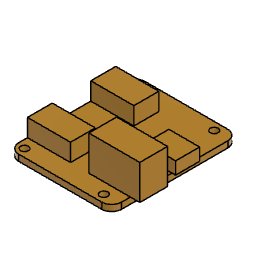
MCP73871 Solar Charger Controller (Autodesk Fusion 360 design; units mm, degrees)
Autodesk Fusion 360 part; units mm, degrees
sketch "Sketch1" plane through (0, 0, 0) normal (0, 0, 1) x (1, 0, 0)
  line L0 (0, 0) -> (33.02, 0)
  line L1 (33.02, 0) -> (33.02, 40.64)
  line L2 (33.02, 40.64) -> (0, 40.64)
  line L3 (0, 40.64) -> (0, 0)
  line L4 (0, 40.64) -> (2.54, 40.64)
  circle A0 centre (2.54, 38.1) radius 1.27
  line L5 (0, 40.64) -> (33.02, 0) construction
  line L6 (33.02, 40.64) -> (0, 0) construction
  line L7 (16.51, 20.32) -> (0, 20.32) construction
  line L8 (16.51, 20.32) -> (16.51, 40.64) construction
  circle A1 centre (2.54, 2.54) radius 1.27
  line L9 (30.46, 38.1) -> (33.02, 38.1) construction
  line L10 (33.02, 38.1) -> (27.94, 38.1) construction
  circle A2 centre (27.94, 38.1) radius 1.27
  circle A3 centre (27.94, 2.54) radius 1.27
  line L11 (0, 40.64) -> (2.54, 40.64)
  line L12 (2.54, 40.64) -> (2.54, 38.1) construction
  line L13 (2.54, 38.1) -> (0, 38.1) construction
  line L14 (0, 38.1) -> (0, 40.64)
  line L15 (27.94, 38.1) -> (33.02, 38.1) construction
  line L16 (33.02, 38.1) -> (33.02, 40.64)
  line L17 (33.02, 40.64) -> (27.94, 40.64)
  line L18 (27.94, 40.64) -> (27.94, 38.1) construction
  line L19 (27.94, 2.54) -> (33.02, 2.54) construction
  line L20 (33.02, 2.54) -> (33.02, 0)
  line L21 (33.02, 0) -> (27.94, 0)
  line L22 (27.94, 0) -> (27.94, 2.54) construction
  line L23 (2.54, 2.54) -> (0, 2.54) construction
  line L24 (0, 2.54) -> (0, 0)
  line L25 (0, 0) -> (2.54, 0)
  line L26 (2.54, 0) -> (2.54, 2.54) construction
  dimension "d1" = 33.02
  dimension "d2" = 40.64
  dimension "d3" = 2.54
  dimension "d5" = 2.54
  dimension "d10" = 5.08
  dimension "d11" = 2.54
  dimension "d16" = 2.54
  constraint horizontal L0
  constraint vertical L1
  constraint horizontal L2
  constraint vertical L3
  constraint coincident L0.start L3.end
  constraint perpendicular L3 L4
  constraint midpoint L5 L7.start
  constraint midpoint L3 L7.end
  constraint midpoint L2 L8.end
  constraint symmetric A0 L7 A1
  constraint coincident L1 L9.end
  constraint perpendicular L1 L9
  constraint parallel L9 L10
  constraint coincident L10.end A2.centre
  constraint symmetric L7 A2 A3
  constraint horizontal L11
  constraint vertical L12
  constraint horizontal L13
  constraint vertical L14
  constraint coincident A0.centre L12.end
  constraint equal L12 L13
  constraint horizontal L15
  constraint vertical L16
  constraint horizontal L17
  constraint vertical L18
  constraint horizontal L19
  constraint vertical L20
  constraint horizontal L21
  constraint vertical L22
  constraint coincident A3.centre L19.start
  constraint horizontal L23
  constraint vertical L24
  constraint horizontal L25
  constraint vertical L26
  constraint coincident A1.centre L23.start
  measures "d1" distance of L0.start L0.end
  measures "d2" distance of L0.start L2.end
  measures "d3" distance of L2.end L4.end
  measures "d5" diameter of A0
  measures "d10" distance of L9.end L10.end
  measures "d11" diameter of A2
  measures "d16" distance of L10.end L17.end
extrude "Extrude1" add sketch "Sketch1" along normal blind 2 contours L0 L1 L2 L3 L4 L11 L14 L16 L17 L20 L21 L24 L25 | A2 | A3 makes body 1
extrude "Extrude2" cut sketch "Sketch1" along normal blind 8.89 contours A2 | A3 bodies 1
fillet "Fillet2" radius 3.175 tangency weight 0.91341 4 edges at (0, 0, 1) (0, 40.64, 1) (33.02, 0, 1) (33.02, 40.64, 1) on bodies 1
ref_plane "WorkPlane1" through (12.7, 20.32, 1) normal (1, 0, 0) x (0, 1, 0)
ref_plane "WorkPlane2" through (16.51, 20.32, 1) normal (0, -1, 0) x (1, 0, 0)
split "Split1" by plane through (12.7, 20.32, 1) normal (1, 0, 0) bodies 1 makes body 2 at (17.5161, 25.9157, 2)
move_body "Move1" bodies 2 to x (1, 0, 0) y (0, 1, 0) z (0, 0, 1) at (7.62, 0, 0)
extrude "Extrude3" add 1 faces at (20.32, 13.5467, 0.6667) along direction (-1, 0, 0) blind 0.19 on bodies 2 bodies 2
move_body "Align1" bodies 1 to x (1, 0, 0) y (0, 1, 0) z (0, 0, 1) at (7.43, 0, 0)
combine "Combine1" operation add target body 1 tool bodies 2
split "Split2" by plane through (16.51, 20.32, 1) normal (0, -1, 0) bodies 1 makes body 3 at (27.6127, 14.7243, 0)
move_body "Move2" bodies 1 to x (1, 0, 0) y (0, 1, 0) z (0, 0, 1) at (0, 15.24, 0)
extrude "Extrude4" add 1 faces at (18.5, 35.56, 1.3333) along direction (0, -1, 0) blind 0.07 on bodies 1 bodies 1
move_body "Align2" bodies 1 to x (1, 0, 0) y (0, 1, 0) z (0, 0, 1) at (0, -15.17, 0)
combine "Combine2" operation add target body 3 tool bodies 1
sketch "Sketch2" plane through (0, 0, 2) normal (0, 0, 1) x (-1, 0, 0)
  circle A0 centre (-35.56, -38.17) radius 1.27
  circle A1 centre (-9.97, -38.17) radius 1.27
  line L0 (-7.43, -37.535) -> (-7.43, -3.175)
  spline S0 degree 3 poles (-10.605, 0) (-10.2204, 0) (-9.8384, -0.0835) (-9.079, -0.3997) (-8.7103, -0.6502) (-8.0884, -1.2692) (-7.8353, -1.6389) (-7.5148, -2.4023) (-7.43, -2.7873) (-7.43, -3.175) knots 0 0 0 0 0.115379 0.115379 0.246087 0.246087 0.377441 0.377441 0.493755 0.493755 0.493755 0.493755
  line L1 (-10.605, 0) -> (-37.465, 0)
  spline S1 degree 3 poles (-40.64, -3.175) (-40.64, -2.7904) (-40.5565, -2.4084) (-40.2403, -1.649) (-39.9898, -1.2803) (-39.3708, -0.6584) (-39.0011, -0.4053) (-38.2377, -0.0848) (-37.8527, 0) (-37.465, 0) knots 0 0 0 0 0.115379 0.115379 0.246087 0.246087 0.377441 0.377441 0.493755 0.493755 0.493755 0.493755
  line L2 (-40.64, -3.175) -> (-40.64, -37.535)
  spline S2 degree 3 poles (-37.465, -40.71) (-37.8496, -40.71) (-38.2316, -40.6265) (-38.991, -40.3103) (-39.3597, -40.0598) (-39.9816, -39.4408) (-40.2347, -39.0711) (-40.5552, -38.3077) (-40.64, -37.9227) (-40.64, -37.535) knots 0 0 0 0 0.115379 0.115379 0.246087 0.246087 0.377441 0.377441 0.493755 0.493755 0.493755 0.493755
  line L3 (-37.465, -40.71) -> (-10.605, -40.71)
  spline S3 degree 3 poles (-7.43, -37.535) (-7.43, -37.9196) (-7.5135, -38.3016) (-7.8297, -39.061) (-8.0802, -39.4297) (-8.6992, -40.0516) (-9.0689, -40.3047) (-9.8323, -40.6252) (-10.2173, -40.71) (-10.605, -40.71) knots 0 0 0 0 0.115379 0.115379 0.246087 0.246087 0.377441 0.377441 0.493755 0.493755 0.493755 0.493755
  circle A2 centre (-35.56, -2.54) radius 1.27
  circle A3 centre (-9.97, -2.54) radius 1.27
  line L4 (-7.43, -6.03) -> (-17.83, -6.03)
  line L5 (-17.83, -6.03) -> (-17.83, -14.98)
  line L6 (-17.83, -14.98) -> (-7.43, -14.98)
  line L7 (-7.43, -6.03) -> (-4.39, -6.03)
  line L8 (-4.39, -6.03) -> (-4.39, -14.98)
  line L9 (-4.39, -14.98) -> (-7.43, -14.98)
  line L10 (-7.43, -14.98) -> (-7.43, -6.03)
  dimension "d24" = 10.4
  dimension "d25" = 8.95
  dimension "d26" = 3.04
  constraint horizontal L4
  constraint vertical L5
  constraint horizontal L6
  constraint coincident L0 L4.start
  constraint horizontal L7
  constraint vertical L8
  constraint horizontal L9
  constraint vertical L10
  measures "d24" distance of L4.start L4.end
  measures "d25" distance of L4.start L6.end
  measures "d26" distance of L4.start L7.end
extrude "Extrude5" add sketch "Sketch2" along normal blind 10.95 separate body contours L0 L4 L5 L6 L10 | L0 L7 L8 L9 L10 makes body 4
sketch "Sketch3" plane through (0, 0, 2) normal (0, 0, 1) x (-1, 0, 0)
  line L0 (-17.83, -14.98) -> (-7.43, -14.98)
  line L1 (-9.7368, -14.98) -> (-9.7368, -19.46)
  line L2 (-7.43, -19.46) -> (-15.4, -19.46)
  line L3 (-15.4, -19.46) -> (-15.4, -27.19)
  line L4 (-15.4, -27.19) -> (-7.43, -27.19)
  line L5 (-7.43, -27.19) -> (-7.43, -19.46)
  line L6 (-7.43, -37.535) -> (-7.43, -3.175)
  line L7 (-7.43, -19.46) -> (-6.26, -19.46)
  line L8 (-6.26, -19.46) -> (-6.26, -27.19)
  line L9 (-6.26, -27.19) -> (-7.43, -27.19)
  line L10 (-7.43, -27.19) -> (-7.43, -19.46)
  dimension "d29" = 4.48
  dimension "d30" = 7.97
  dimension "d31" = 7.73
  dimension "d32" = 1.17
  constraint coincident L0 L1.start
  constraint perpendicular L0 L1
  constraint horizontal L2
  constraint vertical L3
  constraint horizontal L4
  constraint vertical L5
  constraint coincident L2.start L6
  constraint horizontal L7
  constraint vertical L8
  constraint horizontal L9
  constraint vertical L10
  measures "d29" distance of L1.start L1.end
  measures "d30" distance of L2.start L2.end
  measures "d31" distance of L2.start L4.end
  measures "d32" distance of L2.start L7.end
extrude "Extrude6" add sketch "Sketch3" along normal blind 4 contours L2 L3 L4 L5 L6 L10 | L5 L6 L7 L8 L9 L10 bodies 3
sketch "Sketch4" plane through (0, 0, 2) normal (0, 0, 1) x (-1, 0, 0)
  line L0 (-40.64, -3.175) -> (-40.64, -37.535)
  line L1 (-40.64, -6.03) -> (-40.64, -14.09)
  line L2 (-40.64, -6.03) -> (-32.84, -6.03)
  line L3 (-32.84, -6.03) -> (-32.84, -14.03)
  line L4 (-32.84, -14.03) -> (-40.64, -14.03)
  line L5 (-40.64, -14.03) -> (-40.64, -6.03)
  line L6 (-32.84, -14.03) -> (-32.84, -26.47)
  line L7 (-32.84, -26.47) -> (-40.64, -26.47)
  line L8 (-40.64, -26.47) -> (-40.64, -34.53)
  line L9 (-40.64, -34.53) -> (-32.84, -34.53)
  line L10 (-32.84, -34.53) -> (-32.84, -26.47)
  dimension "d35" = 8.06
  dimension "d36" = 7.8
  dimension "d37" = 8
  dimension "d38" = 12.44
  dimension "d39" = 8.06
  constraint coincident L0 L1.start
  constraint horizontal L2
  constraint vertical L3
  constraint horizontal L4
  constraint vertical L5
  constraint vertical L6
  constraint horizontal L7
  constraint vertical L8
  constraint horizontal L9
  constraint vertical L10
  constraint coincident L0 L8.end
  measures "d35" distance of L1.start L1.end
  measures "d36" distance of L1.start L2.end
  measures "d37" distance of L1.start L4.end
  measures "d38" distance of L3.end L6.end
  measures "d39" distance of L6.end L9.end
extrude "Extrude7" add sketch "Sketch4" along normal blind 5.67 separate body contours L0 L1 L2 L3 L4 L5 | L0 L7 L8 L9 L10 makes body 5 at (38.04, 11.3633, 2) makes body 6 at (38.04, 29.1567, 2)
extrude "Extrude8" add 1 faces at (40.64, 8.6967, 3.89) along direction (-1, 0, 0) blind 60.96 on bodies 5 bodies 5 4 3
extrude "Extrude9" add 1 faces at (17.83, 11.68, 11.19) along direction (1, 0, 0) blind 22.8092 on bodies 5 bodies 5
sketch "Sketch5" plane through (40.6392, 0, 0) normal (1, 0, 0) x (0, 1, 0)
  line L0 (6.03, 7.67) -> (14.03, 7.67)
  line L1 (14.03, 7.67) -> (14.03, 2)
  line L2 (14.03, 2) -> (14.98, 2)
  line L3 (14.98, 2) -> (14.98, 12.95)
  line L4 (14.98, 12.95) -> (6.03, 12.95)
  line L5 (6.03, 12.95) -> (6.03, 7.67)
  line L6 (14.98, 2) -> (6.03, 2)
  line L7 (6.03, 2) -> (6.03, 12.95)
  line L8 (6.03, 12.95) -> (14.98, 12.95)
  line L9 (14.98, 12.95) -> (14.98, 2)
  constraint horizontal L6
  constraint vertical L7
  constraint horizontal L8
  constraint vertical L9
  constraint coincident L4.end L5.start
  constraint coincident L2.end L3.start
extrude "Extrude10" add sketch "Sketch5" along normal blind 3.04 bodies 5
extrude "Extrude11" cut 1 faces at (4.39, 11.68, 11.19) along direction (1, 0, 0) blind 22.86 on bodies 5 bodies 5
extrude "Extrude12" cut 1 faces at (-20.32, 8.6967, 3.89) along direction (1, 0, 0) blind 27.7622 on bodies 5 bodies 5
extrude "Extrude13" add 1 faces at (32.84, 31.8433, 3.89) along direction (-1, 0, 0) blind 25.4 on bodies 6 bodies 6 5
extrude "Extrude14" add 1 faces at (6.26, 22.0367, 3.3333) along direction (1, 0, 0) blind 34.3916 separate body on bodies 6 makes body 7
extrude "Extrude15" add 1 faces at (40.6516, 22.0367, 3.3333) along direction (1, 0, 0) blind 1.17 on bodies 7 bodies 7
sketch "Sketch6" plane through (7.44, 0, 0) normal (-1, 0, 0) x (0, -1, 0)
  line L0 (-27.19, 6) -> (-26.47, 6)
  line L1 (-26.47, 6) -> (-26.47, 7.67)
  line L2 (-26.47, 7.67) -> (-34.53, 7.67)
  line L3 (-34.53, 7.67) -> (-34.53, 2)
  line L4 (-34.53, 2) -> (-27.19, 2)
  line L5 (-27.19, 2) -> (-27.19, 6)
  line L6 (-34.53, 2) -> (-26.47, 2)
  line L7 (-26.47, 2) -> (-26.47, 7.67)
  line L8 (-26.47, 7.67) -> (-34.53, 7.67)
  line L9 (-34.53, 7.67) -> (-34.53, 2)
  constraint horizontal L6
  constraint vertical L7
  constraint horizontal L8
  constraint vertical L9
  constraint coincident L1.end L2.start
  constraint coincident L3.end L4.start
extrude "Extrude16" cut 1 faces at (6.26, 22.0367, 3.3333) along direction (1, 0, 0) blind 25.654 on bodies 6 bodies 6 7
extrude "Extrude17" add sketch "Sketch6" against normal blind 24.4856 contours L0 L5 L6 L7 bodies 6 7
sketch "Sketch7" plane through (40.64, 0, 0) normal (1, 0, 0) x (0, 1, 0)
  line L0 (27.19, 2) -> (19.46, 2)
  line L1 (19.46, 2) -> (14.98, 2)
  line L2 (14.98, 2) -> (6.03, 2)
  line L3 (6.03, 2) -> (3.175, 2)
  line L4 (3.175, 0) -> (3.175, 2)
  line L5 (3.175, 0) -> (37.535, 0)
  line L6 (37.535, 2) -> (37.535, 0)
  line L7 (37.535, 2) -> (34.53, 2)
  line L8 (34.53, 2) -> (34.53, 7.67)
  line L9 (34.53, 7.67) -> (26.47, 7.67)
  line L10 (26.47, 7.67) -> (26.47, 6)
  line L11 (26.47, 6) -> (27.19, 6)
  line L12 (27.19, 6) -> (27.19, 2)
  line L13 (34.53, 2) -> (26.47, 2)
  line L14 (26.47, 2) -> (26.47, 7.67)
  line L15 (26.47, 7.67) -> (34.53, 7.67)
  line L16 (34.53, 7.67) -> (34.53, 2)
  constraint horizontal L13
  constraint vertical L14
  constraint horizontal L15
  constraint vertical L16
  constraint coincident L9.end L10.start
  constraint coincident L7.end L8.start
extrude "Extrude18" cut sketch "Sketch7" against normal blind 19.304 contours L8 L9 L10 L11 L12 L13 L14 L15 L16 bodies 6
sketch "Sketch8" plane through (0, 26.47, 0) normal (0, -1, 0) x (1, 0, 0)
  line L0 (21.336, 6) -> (21.336, 7.67)
  line L1 (21.336, 7.67) -> (7.44, 7.67)
  line L2 (7.44, 7.67) -> (7.44, 2)
  line L3 (7.44, 2) -> (31.914, 2)
  line L4 (31.914, 2) -> (31.914, 6)
  line L5 (31.914, 6) -> (21.336, 6)
  line L6 (21.336, 6) -> (31.914, 6)
  line L7 (31.914, 6) -> (31.914, 2)
  line L8 (31.914, 2) -> (21.336, 2)
  line L9 (21.336, 2) -> (21.336, 6)
  constraint horizontal L6
  constraint vertical L7
  constraint horizontal L8
  constraint vertical L9
  constraint coincident L3.end L4.start
  constraint coincident L0.start L5.end
extrude "Extrude19" cut sketch "Sketch8" against normal blind 4.318 contours L3 L4 L5 L6 L7 L8 L9 bodies 6
ref_plane "WorkPlane3" through (21.4122, 10.03, 4.835) normal (-1, 0, 0) x (0, 0, 1)
sketch "Sketch9" plane through (21.4122, 10.03, 4.835) normal (-1, 0, 0) x (0, 1, 0)
extrude "Extrude20" add 1 faces at (32.7264, 9.0133, 12.95) along direction (0, 0, 1) blind 0.254 on bodies 6 bodies 6
ref_plane "WorkPlane4" through (27.25, 10.505, 7.602) normal (-1, 0, 0) x (0, 0, 1)
split "Split3" by plane through (27.25, 10.505, 7.602) normal (-1, 0, 0) bodies 6 makes body 8 at (21.7539, 25.9624, 0)
move_body "Move3" bodies 8 to x (1, 0, 0) y (0, 1, 0) z (0, 0, 1) at (-25.4, 0, 0)
sketch "Sketch10" plane through (1.85, 0, 0) normal (1, 0, 0) x (0, 1, 0)
  line L0 (40.71, 2) -> (14.03, 2)
  line L1 (14.03, 2) -> (14.03, 7.67)
  line L2 (14.03, 7.67) -> (6.03, 7.67)
  line L3 (6.03, 7.67) -> (6.03, 2)
  line L4 (6.03, 2) -> (0, 2)
  line L5 (0, 2) -> (0, 0)
  line L6 (0, 0) -> (40.71, 0)
  line L7 (40.71, 0) -> (40.71, 2)
  line L8 (6.03, 2) -> (14.03, 2)
  line L9 (14.03, 2) -> (14.03, 7.67)
  line L10 (14.03, 7.67) -> (6.03, 7.67)
  line L11 (6.03, 7.67) -> (6.03, 2)
  constraint horizontal L8
  constraint vertical L9
  constraint horizontal L10
  constraint vertical L11
  constraint coincident L1.end L2.start
  constraint coincident L3.end L4.start
extrude "Extrude21" cut sketch "Sketch10" against normal blind 5.9182 contours L1 L2 L3 L8 L9 L10 L11 bodies 8
move_body "Align3" bodies 8 to x (1, 0, 0) y (0, 1, 0) z (0, 0, 1) at (25.4, 0, 0)
combine "Combine6" operation add target body 8 tool bodies 6
combine "Combine3" [suppressed]
combine "Combine4" [suppressed]
combine "Combine5" [suppressed]
